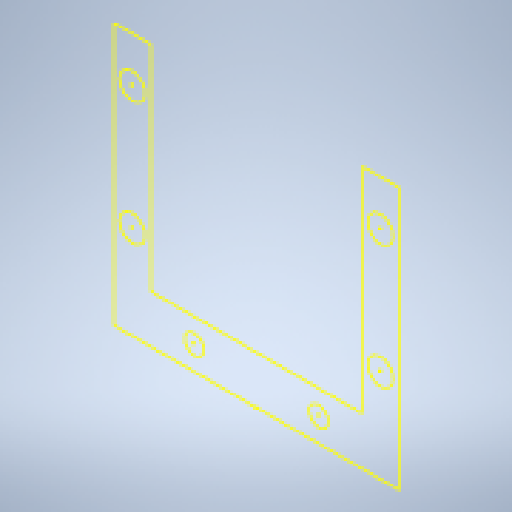
# Autodesk Inventor part: Mounting Bar
Saved by Autodesk Inventor 2023.1 (Build 271208000, 208)
## iProperties
Created: 2022-08-13
Part Number: Mounting Bar
Material: Generic
Document SubType Name: Modeling
Designer: xSibe
Density: 1 g/cm^3
Appearance: Steel - Polished
Author: xSibe
Autodesk Inventor part; units mm, degrees
ref_plane "YZ Plane" through (0, 0, 0) normal (1, 0, 0) x (0, 1, 0)
ref_plane "XZ Plane" through (0, 0, 0) normal (0, 1, 0) x (-1, 0, 0)
ref_plane "XY Plane" through (0, 0, 0) normal (0, 0, 1) x (1, 0, 0)
sketch "Sketch1" plane through (0, 0, 0) normal (0, 0, 1) x (1, 0, 0)
  line L0 (22.9, 0.025) -> (-22.9, 0.025) projected
  line L1 (22.9, 42.1) -> (22.9, 0.025) projected
  line L2 (22.9, 42.1) -> (17.05, 42.1) projected
  line L3 (17.05, 7.7) -> (17.05, 42.1) projected
  line L4 (-17.05, 7.7) -> (17.05, 7.7) projected
  line L5 (-17.05, 7.7) -> (-17.05, 42.1) projected
  line L6 (-17.05, 42.1) -> (-22.9, 42.1) projected
  line L7 (-22.9, 0.025) -> (-22.9, 42.1) projected
  circle A0 centre (19.9, 34.8) radius 2.0625 projected
  circle A1 centre (-19.9, 34.8) radius 2.0625 projected
  circle A2 centre (19.9, 15) radius 2.0625 projected
  circle A3 centre (-19.9, 15) radius 2.0625 projected
  circle A4 centre (10, 3.85) radius 1.5625 projected
  circle A5 centre (-10, 3.85) radius 1.5625 projected
  point P0 (0, 0)
extrude "Extrusion1" add sketch "Sketch1" along normal mid plane 49.8 contours A4 | A5
body "Solid1"
